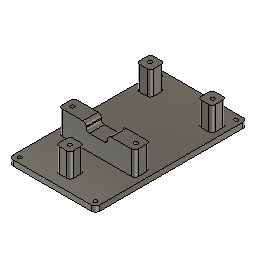
Bottom Housing v4 (Autodesk Fusion 360 design; units mm, degrees)
Autodesk Fusion 360 part; units mm, degrees
note: some values were not read from the file. Set by a fixed rule: which sketch regions a step uses.
sketch "Sketch2" plane through (0, 0, 0) normal (0, 0, 1) x (-1, 0, 0)
  line L0 (29.6528, -57.1307) -> (30.0921, -57.0728)
  line L1 (30.0921, -57.0728) -> (30.5248, -56.9769)
  line L2 (30.5248, -56.9769) -> (30.9475, -56.8436)
  line L3 (30.9475, -56.8436) -> (31.3569, -56.674)
  line L4 (31.3569, -56.674) -> (31.75, -56.4694)
  line L5 (31.75, -56.4694) -> (32.1238, -56.2313)
  line L6 (32.1238, -56.2313) -> (32.4754, -55.9615)
  line L7 (32.4754, -55.9615) -> (32.8021, -55.6621)
  line L8 (32.8021, -55.6621) -> (33.1015, -55.3354)
  line L9 (33.1015, -55.3354) -> (33.3713, -54.9838)
  line L10 (33.3713, -54.9838) -> (33.6094, -54.61)
  line L11 (33.6094, -54.61) -> (33.814, -54.2169)
  line L12 (33.814, -54.2169) -> (33.9836, -53.8075)
  line L13 (33.9836, -53.8075) -> (34.1169, -53.3848)
  line L14 (34.1169, -53.3848) -> (34.2128, -52.9521)
  line L15 (34.2128, -52.9521) -> (34.2707, -52.5128)
  line L16 (34.2707, -52.5128) -> (34.29, -52.07)
  line L17 (34.29, -52.07) -> (34.29, 52.07)
  line L18 (34.29, 52.07) -> (34.2707, 52.5128)
  line L19 (34.2707, 52.5128) -> (34.2128, 52.9521)
  line L20 (34.2128, 52.9521) -> (34.1169, 53.3848)
  line L21 (34.1169, 53.3848) -> (33.9836, 53.8075)
  line L22 (33.9836, 53.8075) -> (33.814, 54.2169)
  line L23 (33.814, 54.2169) -> (33.6094, 54.61)
  line L24 (33.6094, 54.61) -> (33.3713, 54.9838)
  line L25 (33.3713, 54.9838) -> (33.1015, 55.3354)
  line L26 (33.1015, 55.3354) -> (32.8021, 55.6621)
  line L27 (32.8021, 55.6621) -> (32.4754, 55.9615)
  line L28 (32.4754, 55.9615) -> (32.1238, 56.2313)
  line L29 (32.1238, 56.2313) -> (31.75, 56.4694)
  line L30 (31.75, 56.4694) -> (31.3569, 56.674)
  line L31 (31.3569, 56.674) -> (30.9475, 56.8436)
  line L32 (30.9475, 56.8436) -> (30.5248, 56.9769)
  line L33 (30.5248, 56.9769) -> (30.0921, 57.0728)
  line L34 (30.0921, 57.0728) -> (29.6528, 57.1307)
  line L35 (29.6528, 57.1307) -> (29.21, 57.15)
  line L36 (29.21, 57.15) -> (-29.21, 57.15)
  line L37 (-29.21, 57.15) -> (-29.6528, 57.1307)
  line L38 (-29.6528, 57.1307) -> (-30.0921, 57.0728)
  line L39 (-30.0921, 57.0728) -> (-30.5248, 56.9769)
  line L40 (-30.5248, 56.9769) -> (-30.9475, 56.8436)
  line L41 (-30.9475, 56.8436) -> (-31.3569, 56.674)
  line L42 (-31.3569, 56.674) -> (-31.75, 56.4694)
  line L43 (-31.75, 56.4694) -> (-32.1238, 56.2313)
  line L44 (-32.1238, 56.2313) -> (-32.4754, 55.9615)
  line L45 (-32.4754, 55.9615) -> (-32.8021, 55.6621)
  line L46 (-32.8021, 55.6621) -> (-33.1015, 55.3354)
  line L47 (-33.1015, 55.3354) -> (-33.3713, 54.9838)
  line L48 (-33.3713, 54.9838) -> (-33.6094, 54.61)
  line L49 (-33.6094, 54.61) -> (-33.814, 54.2169)
  line L50 (-33.814, 54.2169) -> (-33.9836, 53.8075)
  line L51 (-33.9836, 53.8075) -> (-34.1169, 53.3848)
  line L52 (-34.1169, 53.3848) -> (-34.2128, 52.9521)
  line L53 (-34.2128, 52.9521) -> (-34.2707, 52.5128)
  line L54 (-34.2707, 52.5128) -> (-34.29, 52.07)
  line L55 (-34.29, 52.07) -> (-34.29, -52.07)
  line L56 (-34.29, -52.07) -> (-34.2707, -52.5128)
  line L57 (-34.2707, -52.5128) -> (-34.2128, -52.9521)
  line L58 (-34.2128, -52.9521) -> (-34.1169, -53.3848)
  line L59 (-34.1169, -53.3848) -> (-33.9836, -53.8075)
  line L60 (-33.9836, -53.8075) -> (-33.814, -54.2169)
  line L61 (-33.814, -54.2169) -> (-33.6094, -54.61)
  line L62 (-33.6094, -54.61) -> (-33.3713, -54.9838)
  line L63 (-33.3713, -54.9838) -> (-33.1015, -55.3354)
  line L64 (-33.1015, -55.3354) -> (-32.8021, -55.6621)
  line L65 (-32.8021, -55.6621) -> (-32.4754, -55.9615)
  line L66 (-32.4754, -55.9615) -> (-32.1238, -56.2313)
  line L67 (-32.1238, -56.2313) -> (-31.75, -56.4694)
  line L68 (-31.75, -56.4694) -> (-31.3569, -56.674)
  line L69 (-31.3569, -56.674) -> (-30.9475, -56.8436)
  line L70 (-30.9475, -56.8436) -> (-30.5248, -56.9769)
  line L71 (-30.5248, -56.9769) -> (-30.0921, -57.0728)
  line L72 (-30.0921, -57.0728) -> (-29.6528, -57.1307)
  line L73 (-29.6528, -57.1307) -> (-29.21, -57.15)
  line L74 (-29.21, -57.15) -> (29.21, -57.15)
  line L75 (29.21, -57.15) -> (29.6528, -57.1307)
  circle A0 centre (26.67, 50.025) radius 0.7
  circle A1 centre (20.32, 50.025) radius 0.7
  circle A2 centre (26.67, 33.795) radius 0.7
  circle A3 centre (20.32, 33.795) radius 0.7
  circle A4 centre (13.97, 50.025) radius 0.7
  circle A5 centre (13.97, 33.795) radius 0.7
  circle A6 centre (5.13, 26.87) radius 1.15
  circle A7 centre (29.21, 19.05) radius 1.75
  circle A8 centre (5.13, 22.17) radius 1.15
  circle A9 centre (5.13, 17.47) radius 1.15
  circle A10 centre (-0.1534, 50.7401) radius 1.75
  circle A11 centre (-14.15, 50.025) radius 0.7
  circle A12 centre (-0.17, 26.87) radius 1.15
  circle A13 centre (-5.47, 26.87) radius 1.15
  circle A14 centre (-14.15, 33.795) radius 0.7
  circle A15 centre (-20.5, 50.025) radius 0.7
  circle A16 centre (-26.85, 50.025) radius 0.7
  circle A17 centre (-20.5, 33.795) radius 0.7
  circle A18 centre (-26.85, 33.795) radius 0.7
  circle A19 centre (-0.17, 22.17) radius 1.15
  circle A20 centre (-5.47, 22.17) radius 1.15
  circle A21 centre (-0.17, 17.47) radius 1.15
  circle A22 centre (-5.47, 17.47) radius 1.15
  circle A23 centre (-0.17, 3.81) radius 0.45
  circle A24 centre (-0.17, 1.27) radius 0.45
  circle A25 centre (-29.21, 19.05) radius 1.75
  circle A26 centre (31.724, -24.1849) radius 0.45
  circle A27 centre (29.184, -24.1849) radius 0.45
  circle A28 centre (26.67, -36.505) radius 0.55
  circle A29 centre (24.13, -36.505) radius 0.55
  circle A30 centre (21.59, -36.505) radius 0.55
  circle A31 centre (29.21, -52.07) radius 1.75
  circle A32 centre (21.59, -44.45) radius 0.5
  circle A33 centre (19.05, -44.45) radius 0.5
  circle A34 centre (11.43, -44.45) radius 0.5
  circle A35 centre (8.89, -44.45) radius 0.5
  circle A36 centre (-13.105, -19.09) radius 0.4
  circle A37 centre (-17.985, -19.09) radius 0.4
  circle A38 centre (-0.205, -41.91) radius 0.5
  circle A39 centre (-2.745, -41.91) radius 0.5
  circle A40 centre (-5.285, -41.91) radius 0.5
  circle A41 centre (-29.21, -52.07) radius 1.75
  circle A42 centre (29.21, 19.05) radius 1.75
  circle A43 centre (-0.1534, 50.7401) radius 1.75
  circle A44 centre (-29.21, 19.05) radius 1.75
  circle A45 centre (29.21, -52.07) radius 1.75
  circle A46 centre (-29.21, -52.07) radius 1.75
  line L76 (-40.1186, 67.15) -> (39.8814, 67.15)
  line L77 (39.8814, 67.15) -> (39.8814, -72.85)
  line L78 (39.8814, -72.85) -> (-40.1186, -72.85)
  line L79 (-40.1186, -72.85) -> (-40.1186, 67.15)
  line L80 (-35.1186, -67.85) -> (-35.1186, 62.15)
  line L81 (-35.1186, 62.15) -> (34.8814, 62.15)
  line L82 (34.8814, 62.15) -> (34.8814, -67.85)
  line L83 (34.8814, -67.85) -> (-35.1186, -67.85)
  circle A47 centre (-35.1186, 62.15) radius 1.65
  circle A48 centre (34.8814, 62.15) radius 1.65
  circle A49 centre (34.8814, -67.85) radius 1.65
  circle A50 centre (-35.1186, -67.85) radius 1.65
  line L84 (-35.1186, 25.7548) -> (35.1185, 25.7548)
  line L85 (35.1185, 25.7548) -> (35.1185, 11.7548)
  line L86 (35.1185, 11.7548) -> (-35.1186, 11.7548)
  line L87 (-35.1186, 11.7548) -> (-35.1186, 25.7548)
  line L88 (-0.1186, 67.15) -> (-0.1186, -72.85) construction
  line L89 (-10.1186, 25.7548) -> (-10.1186, 11.7548)
  line L90 (9.8814, 25.7548) -> (9.8814, 11.7548)
  line L91 (-35.1186, -45.5115) -> (-22.1186, -45.5115)
  line L92 (-22.1186, -45.5115) -> (-22.1186, -58.5115)
  line L93 (-22.1186, -58.5115) -> (-35.1186, -58.5115)
  line L94 (-35.1186, -58.5115) -> (-35.1186, -45.5115)
  line L95 (21.8814, -45.5115) -> (21.8814, -58.5115)
  line L96 (34.8814, -45.5115) -> (21.8814, -45.5115)
  line L97 (21.8814, -58.5115) -> (34.8814, -58.5115)
  line L98 (-6.6186, 57.15) -> (6.3814, 57.15)
  line L99 (6.3814, 57.15) -> (6.3814, 44.15)
  line L100 (6.3814, 44.15) -> (-6.6186, 44.15)
  line L101 (-6.6186, 44.15) -> (-6.6186, 57.15)
  dimension "d1" = 80
  dimension "d2" = 140
  dimension "d4" = 5
  dimension "d6" = 3.3
  dimension "d7" = 3.3
  dimension "d8" = 3.3
  dimension "d9" = 3.3
  dimension "d11" = 14
  dimension "d12" = 10
  dimension "d13" = 13
  dimension "d14" = 13
  dimension "d15" = 13
  dimension "d16" = 13
  dimension "d35" = 10
  constraint concentric A7 A42
  constraint concentric A10 A43
  constraint concentric A25 A44
  constraint concentric A31 A45
  constraint concentric A41 A46
  constraint horizontal L76
  constraint vertical L77
  constraint horizontal L78
  constraint vertical L79
  constraint coincident L80.end L81.start
  constraint coincident L81.end L82.start
  constraint coincident L82.end L83.start
  constraint coincident L80.start L83.end
  constraint horizontal L84
  constraint vertical L85
  constraint horizontal L86
  constraint vertical L87
  constraint coincident L80 L84.start
  constraint midpoint L76 L88.start
  constraint midpoint L78 L88.end
  constraint coincident L84 L89.start
  constraint coincident L86 L89.end
  constraint perpendicular L86 L89
  constraint symmetric L88 L89.start L90.start
  constraint symmetric L88 L89.end L90.end
  constraint horizontal L91
  constraint vertical L92
  constraint horizontal L93
  constraint vertical L94
  constraint coincident L80 L91.start
  constraint symmetric L88 L91.start L96.start
  constraint symmetric L88 L91.end L95.start
  constraint symmetric L88 L92.end L95.end
  constraint symmetric L88 L93.end L97.end
  constraint horizontal L98
  constraint vertical L99
  constraint horizontal L100
  constraint vertical L101
  constraint coincident L36 L98.start
  constraint symmetric L88 L99 L101
  measures "d1" distance of L76.start L76.end
  measures "d2" distance of L76.start L78.end
  measures "d6" diameter of A47
  measures "d7" diameter of A48
  measures "d8" diameter of A49
  measures "d9" diameter of A50
  measures "d11" distance of L84.start L86.end
  measures "d12" distance of L88 L90
  measures "d13" distance of L91.start L91.end
  measures "d14" distance of L91.start L93.end
  measures "d15" distance of L98.start L98.end
  measures "d16" distance of L98.start L100.end
  measures "d35" distance of L36 L76
extrude "Extrude1" add sketch "Sketch2" along normal blind 5 contours L0 L1 L2 L3 L4 L5 L6 L7 L8 L9 L10 L11 L12 L13 L14 L15 L16 L17 L74 L75 L95 L96 | L0 L1 L2 L3 L4 L5 L6 L7 L8 L9 L10 L11 L12 L13 L14 L15 L16 L17 L74 L75 L82 L95 L96 L97 | L74 L80 L82 L83 A49 A50 L92 L93 L95 L97 | L17 L55 L74 L86 L91 L92 L95 L96 | L55 L56 L57 L58 L59 L60 L61 L62 L63 L64 L65 L66 L67 L68 L69 L70 L71 L72 L73 L74 L80 L91 L92 L93 L94 | L55 L56 L57 L58 L59 L60 L61 L62 L63 L64 L65 L66 L67 L68 L69 L70 L71 L72 L73 L74 L91 L92 | L17 L82 L86 L96 | L55 L80 L86 L91 | L17 L84 L86 L90 | L17 L82 L84 L86 | L55 L80 L84 L86 L87 | L55 L84 L86 L89 | L17 L18 L19 L20 L21 L22 L23 L24 L25 L26 L27 L28 L29 L30 L31 L32 L33 L34 L35 L36 L37 L38 L39 L40 L41 L42 L43 L44 L45 L46 L47 L48 L49 L50 L51 L52 L53 L54 L55 A6 A12 A13 L84 L99 L100 L101 | L17 L18 L19 L20 L21 L22 L23 L24 L25 L26 L27 L28 L29 L30 L31 L32 L33 L34 L35 L36 L37 L38 L39 L40 L41 L42 L43 L44 L45 L46 L47 L48 L49 L50 L51 L52 L53 L54 L55 L80 L81 L82 A47 A48 L84 L98 | L82 L84 L85 L86 | A6 A12 A13 L84 L86 L89 L90 | A6 L84 | A6 L84 | A13 L84 | A13 L84 | A12 L84 | A12 L84 | L36 L98 L99 L100 L101 | A0 | A1 | A2 | A3 | A4 | A5 | A8 | A9 | A11 | A14 | A15 | A16 | A17 | A18 | A19 | A20 | A21 | A22 | A23 | A24 | A26 | A27 | A28 | A29 | A30 | A32 | A33 | A34 | A35 | A36 | A37 | A38 | A39 | A40 | L76 L77 L78 L79
extrude "Extrude2" add sketch "Sketch2" along normal blind 27 contours L0 L1 L2 L3 L4 L5 L6 L7 L8 L9 L10 L11 L12 L13 L14 L15 L16 L17 L74 L75 L95 L96 | L0 L1 L2 L3 L4 L5 L6 L7 L8 L9 L10 L11 L12 L13 L14 L15 L16 L17 L74 L75 L82 L95 L96 L97 | L55 L56 L57 L58 L59 L60 L61 L62 L63 L64 L65 L66 L67 L68 L69 L70 L71 L72 L73 L74 L80 L91 L92 L93 L94 | L55 L56 L57 L58 L59 L60 L61 L62 L63 L64 L65 L66 L67 L68 L69 L70 L71 L72 L73 L74 L91 L92 | L17 L84 L86 L90 | L17 L82 L84 L86 | L55 L80 L84 L86 L87 | L55 L84 L86 L89 | L82 L84 L85 L86 | L36 L98 L99 L100 L101
fillet "Fillet1" radius 3 2 edges at (-34.8814, 58.5115, 16) (35.1186, 58.5115, 16)
fillet "Fillet1" radius 3 6 edges at (35.1186, 45.5115, 16) (22.1186, 45.5115, 16) (22.1186, 58.5115, 16) (-21.8814, 45.5115, 16) (-21.8814, 58.5115, 16) (-34.8814, 45.5115, 16)
fillet "Fillet1" radius 3 4 edges at (6.6186, -44.15, 16) (6.6186, -57.15, 16) (-6.3814, -44.15, 16) (-6.3814, -57.15, 16)
fillet "Fillet2" radius 4 4 edges at (40.1186, 72.85, 2.5) (-39.8814, 72.85, 2.5) (40.1186, -67.15, 2.5) (-39.8814, -67.15, 2.5)
extrude "Extrude3" add sketch "Sketch2" along normal blind 20 contours A6 A12 A13 L84 L86 L89 L90 | A6 L84 | A13 L84 | A12 L84 | A8 | A9 | A19 | A20 | A21 | A22 picked at (5.0829, 25.7461) picked at (-5.5171, 25.7461) picked at (-0.2171, 25.7461)
fillet "Fillet3" radius 3 4 edges at (-9.8814, -18.7548, 20) (-9.8814, -18.7548, 27) (10.1186, -18.7548, 27) (10.1186, -18.7548, 20)
fillet "Fillet4" radius 3 4 edges at (35.1186, -25.7548, 16) (35.1186, -11.7548, 16) (-35.1185, -25.7548, 16) (-35.1185, -11.7548, 16)
